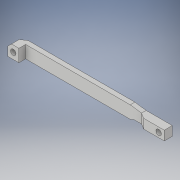
# Autodesk Inventor part: Abzugstange
Saved by Autodesk Inventor 2019 (Build 230136000, 136)
## iProperties
Created: 2021-03-08
Part Number: Abzugstange
Material: Generic
Document SubType Name: Modeling
Designer: Lukas
Density: 1 g/cm^3
Appearance: Default
Author: Lukas
Autodesk Inventor part; units mm, degrees
ref_plane "YZ Plane" through (0, 0, 0) normal (1, 0, 0) x (0, 1, 0)
ref_plane "XZ Plane" through (0, 0, 0) normal (0, 1, 0) x (-1, 0, 0)
ref_plane "XY Plane" through (0, 0, 0) normal (0, 0, 1) x (1, 0, 0)
sketch "Sketch1" plane through (0, 0, 0) normal (0, 0, 1) x (1, 0, 0)
  line L0 (-41, -3.35) -> (21, -3.35)
  line L1 (41, -2.5) -> (41, 2.5)
  line L2 (21, 3.35) -> (-41, 3.35)
  line L3 (-41, 3.35) -> (-41, -3.35)
  circle A0 centre (-38, 0) radius 1.45
  line L4 (21, -3.35) -> (23, -2.5)
  line L5 (23, -2.5) -> (41, -2.5)
  line L6 (21, 3.35) -> (27, 2.5)
  line L7 (27, 2.5) -> (41, 2.5)
  point P0 (0, 0)
  point P1 (41, 0)
  point P2 (-41, 0)
  dimension "d4" = 2.9
  dimension "d5" = 3
  dimension "d29" = 82
  dimension "d30" = 6.7
  dimension "d31" = 5
  dimension "d32" = 18
  dimension "d33" = 14
  dimension "d34" = 2
  dimension "d35" = 6
  dimension "d36" = 41
  constraints: 16 end point, 3 horizontal alignment, 2 horizontal, 2 midpoint, 2 parallel, 2 perpendicular, 1 centre point
  measures "d4" diameter of A0
  measures "d5" distance from line of L3 A0.centre
  measures "d29" distance between parallel lines of L3 L1
  measures "d30" distance of L2.end L0.start
  measures "d31" distance of L1.start L1.end
  measures "d32" distance of L4.end L1.start
  measures "d33" distance of L6.end L1.end
  measures "d34" horizontal distance of L4.end L0.end
  measures "d35" horizontal distance of L2.start L6.end
  measures "d36" distance from line of point (0, 0) L3
extrude "Extrusion1" add sketch "Sketch1" along normal blind 2.5
sketch "Sketch2" plane through (0, 0, 2.5) normal (0, 0, 1) x (1, 0, 0)
  circle A0 centre (-38, 0) radius 1.45 projected
  line L0 (-41, -3.35) -> (21, -3.35) projected
  line L1 (41, -2.5) -> (41, 2.5) projected
  line L2 (21, 3.35) -> (-41, 3.35) projected
  line L3 (-41, 3.35) -> (-41, -3.35) projected
  line L4 (-35, 3.35) -> (-35, -3.35)
  line L5 (21, -3.35) -> (23, -2.5) projected
  line L6 (23, -2.5) -> (41, -2.5) projected
  line L7 (41, 2.5) -> (27, 2.5) projected
  line L8 (27, 2.5) -> (21, 3.35) projected
  point P0 (0, 0)
  dimension "d6" = 6
  constraints: 2 end point, 2 point on line, 1 perpendicular
  measures "d6" distance between parallel lines of L3 L4
extrude "Extrusion2" add sketch "Sketch2" along normal blind 3.6 contours L3 L2 L4 L0
chamfer "Chamfer7" distance 2 angle 45 1 edges at (-41, 3.35, 3.05)
chamfer "Chamfer8" distance 2 angle 45 1 edges at (-40, 2.35, 0)
sketch "Sketch3" plane through (27, 2.5, 0) normal (0, 1, 0) x (1, 0, 0)
  line L0 (14, 0) -> (0, 0) projected
  line L1 (0, 0) -> (0, -2.5) projected
  line L2 (14, -2.5) -> (0, -2.5) projected
  line L3 (14, 0) -> (14, -2.5) projected
  line L4 (14, -4.3) -> (3, -4.3)
  line L5 (14, -2.5) -> (0, -2.5) projected
  line L6 (3, -4.3) -> (0, -2.5)
  line L7 (14, -2.5) -> (14, -4.3)
  point P0 (-27, 0)
  dimension "d48" = 3
  dimension "d51" = 1.8
  constraints: 6 end point, 1 horizontal, 1 perpendicular, 1 point on line
  measures "d48" distance from line of L1 L4.end
  measures "d51" distance between parallel lines of L4 L2
extrude "Extrusion3" add sketch "Sketch3" against normal up to surface (5 mm away) contours L7 L4 L6 L2
sketch "Sketch4" plane through (0, 0, 0) normal (0, 0, -1) x (-1, 0, 0)
  circle A0 centre (-38, 0) radius 1.45
  line L0 (-41, -2.5) -> (-41, 2.5) projected
  point P0 (0, 0)
  dimension "d52" = 3
  dimension "d53" = 2.9
  constraints: 1 centre point, 1 horizontal alignment
  measures "d52" distance from line of A0.centre L0
  measures "d53" diameter of A0
extrude "Extrusion4" cut sketch "Sketch4" against normal through all
equation "\"d36\" = 0.5 * d29"
body "Solid1"
